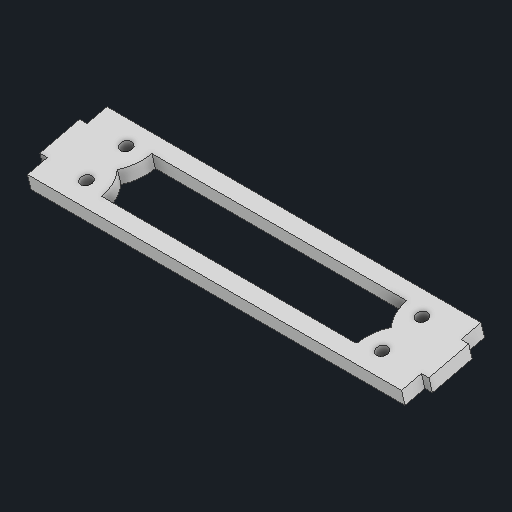
# Autodesk Inventor part: motor_mount
Saved by Autodesk Inventor 2023 (Build 270158030, 158C)
## iProperties
Created: 2022-03-25
Part Number: motor_mount
Material: Generic
Document SubType Name: Modeling
Designer: kardo
Density: 1 g/cm^3
Appearance: Default
Author: kardo
Autodesk Inventor part; units mm, degrees
ref_plane "YZ Plane" through (0, 0, 0) normal (1, 0, 0) x (0, 1, 0)
ref_plane "XZ Plane" through (0, 0, 0) normal (0, 1, 0) x (-1, 0, 0)
ref_plane "XY Plane" through (0, 0, 0) normal (0, 0, 1) x (1, 0, 0)
derived "parameters_frame.ipt"
derived "stencil_frame.ipt"
sketch "sk_cowl_joint_locations" plane through (54.6, 0, 0) normal (1, 0, 0) x (0, 1, 0)
  line L0 (-345, 16.32) -> (-262.2001, 18.586) construction
  arc A0 (-262.2001, 18.586) -> (-241.5001, 19.2432) centre (-326.8578, 2381.2399) ccw construction
  line L1 (-241.5001, 19.2432) -> (11.22, 28.376) construction
  arc A1 (36.465, 28.832) -> (11.22, 28.376) centre (36.465, -670.197) ccw construction
  line L2 (36.465, 28.832) -> (112.2, 28.832) construction
  line L3 (94.8, 30.032) -> (36.465, 30.032) construction
  arc A2 (36.465, 30.032) -> (11.1767, 29.5752) centre (36.465, -670.197) ccw construction
  line L4 (11.1767, 29.5752) -> (-241.5434, 20.4424) construction
  arc A3 (-262.2329, 19.7855) -> (-241.5434, 20.4424) centre (-326.8578, 2381.2399) ccw construction
  line L5 (-262.2329, 19.7855) -> (-345, 17.5204) construction
  line L6 (-230.0001, 3089.1136) -> (-230.0001, -1866.0023) construction
  line L7 (-114.9999, 3089.1136) -> (-114.9999, -1866.0023) construction
  line L8 (-345, 3089.1136) -> (-345, -1866.0023) construction
  line L9 (0, 3089.1136) -> (0, -1866.0023) construction
  line L10 (-230.0001, 45.0685) -> (-230.0001, 20.8596) construction
  line L11 (-114.9999, 49.9659) -> (-114.9999, 25.0155) construction
  line L12 (-345, 17.5204) -> (-345, 17.5204)
  line L13 (-345, 17.5204) -> (-345, 36.9221) construction
  line L14 (-844.2225, 3013.4797) -> (331.7536, -1884.8132) construction
  line L15 (-344.7623, 36.9221) -> (-345, 39.712) construction
  line L16 (0, 51.6) -> (0, 29.1713) construction
  line L17 (-135.791, 45.5154) -> (-130.7328, 24.4469) construction
  line L18 (-128.1079, 30.6478) -> (-131.9974, 29.714) construction
  line L19 (-130.6369, 41.1821) -> (-134.5264, 40.2483) construction
  spline S0 degree 2 poles (-345, 39.712) (-172.656, 54.3934) (0, 54.4) knots 0 0 0 1 1 1
  spline S1 degree 3 poles (0, 54.4) (37.026, 54.4) (80.784, 47.9917) (112.2, 37.536) knots 1 1 1 1 2 2 2 2
  spline S2 degree 3 poles (111.3158, 34.8793) (106.1488, 36.5989) (96.4909, 39.4217) (84.5445, 42.2265) (75.2974, 44.1359) (69.0059, 45.3094) (61.0256, 46.6466) (54.5653, 47.6105) (46.4371, 48.6777) (39.9092, 49.4192) (31.7597, 50.2005) (25.2653, 50.7072) (17.2211, 51.1873) (9.2717, 51.5118) (3.0586, 51.6) (0, 51.6) knots 1 1 1 1 1.166667 1.291667 1.333333 1.416667 1.458333 1.541667 1.583333 1.666667 1.708333 1.791667 1.833333 1.916667 2 2 2 2
  spline S3 degree 3 poles (0, 51.6) (-19.1708, 51.5993) (-52.7146, 51.3604) (-91.0402, 50.6121) (-119.7801, 49.8472) (-138.9379, 49.2354) (-162.8824, 48.3434) (-182.0358, 47.528) (-205.975, 46.3814) (-225.1241, 45.3623) (-249.0578, 43.9611) (-268.2026, 42.7383) (-292.131, 41.0825) (-316.0566, 39.2994) (-335.1942, 37.7372) (-344.7623, 36.9221) knots 0 0 0 0 0.166667 0.291667 0.333333 0.416667 0.458333 0.541666 0.583333 0.666666 0.708333 0.791666 0.833333 0.916666 1 1 1 1
  line L20 (-135.791, 45.5154) -> (-131.9015, 46.4492) construction
  line L21 (-130.7328, 24.4469) -> (-126.8434, 25.3807) construction
  line L22 (-131.9015, 46.4492) -> (-132.0904, 52.2462) construction
  point P0 (0, 0)
  point P1 (-345, 27.2213)
  point P2 (-230.0001, 32.964)
  point P3 (-114.9999, 37.4907)
  point P4 (0, 40.3857)
  point P5 (0, 40.3857)
ref_plane "plane_motor_mount" through (0, -120.75, 0) normal (0, 0.9723699, 0.2334454) x (-1, 0, 0)
ref_plane "plane_cowl_right" through (54.6, 0, 0) normal (1, 0, 0) x (0, 1, 0)
ref_plane "plane_symmetry" through (0, 0, 0) normal (1, 0, 0) x (0, 1, 0)
sketch "sk_base" plane through (0, -120.75, 0) normal (0, 0.9723699, 0.2334454) x (-1, 0, 0)
  line L0 (-54.6, -1321.492) -> (-54.6, 2983.6601) construction
  line L1 (0, -1321.492) -> (0, 2983.6601) projected
  line L2 (0, 47.7691) -> (-49.6, 47.7691)
  line L3 (-49.6, 47.7691) -> (-49.6, 42.3523)
  line L4 (-49.6, 42.3523) -> (-51.6, 42.3523)
  line L5 (-51.6, 42.3523) -> (-51.6, 31.5187)
  line L6 (-51.6, 31.5187) -> (-49.6, 31.5187)
  line L7 (-49.6, 31.5187) -> (-49.6, 26.1019)
  line L8 (-49.6, 26.1019) -> (0, 26.1019)
  point P0 (0, -28.1885)
  point P1 (-54.6, 42.3523)
  point P2 (-54.6, 31.5187)
  point P3 (-54.6, 47.7691)
  point P4 (-54.6, 26.1019)
  dimension "d2" = 5
  dimension "d3" = 2
  constraints: 14 end point, 6 point on line, 4 perpendicular, 2 parallel, 1 collinear
  measures "d2" distance between parallel lines of L0 L3
  measures "d3" distance between parallel lines of L3 L5
extrude "thicken" add sketch "sk_base" against normal blind 4
sketch "sk_cut" plane through (0, -120.75, 0) normal (0, 0.9723699, 0.2334454) x (-1, 0, 0)
  line L0 (-49.6, 26.1019) -> (0, 26.1019) construction
  line L1 (0, 26.1019) -> (0, 47.7691) projected
  line L2 (0, 47.7691) -> (-49.6, 47.7691) construction
  line L3 (-49.6, 47.7691) -> (-49.6, 42.3523) construction
  line L4 (-49.6, 42.3523) -> (-51.6, 42.3523) construction
  line L5 (-51.6, 42.3523) -> (-51.6, 31.5187) construction
  line L6 (-51.6, 31.5187) -> (-49.6, 31.5187) construction
  line L7 (-49.6, 31.5187) -> (-49.6, 26.1019) construction
  line L8 (0, 26.1019) -> (0, 47.7691) projected
  line L9 (0, 43.7691) -> (-33.8, 43.7691)
  line L10 (0, 30.1019) -> (-33.8, 30.1019)
  arc A0 (-33.8, 30.1019) -> (-36.2872, 36.9355) centre (-44.4312, 30.1019) ccw
  arc A1 (-36.2872, 36.9355) -> (-33.8, 43.7691) centre (-44.4312, 43.7691) ccw
  circle A2 centre (-39.2, 42.3691) radius 1.5
  circle A3 centre (-39.2, 31.5019) radius 1.5
  line L11 (-44.6, 47.7691) -> (-44.6, 26.1019) construction
  line L12 (-33.8, 43.7691) -> (-33.8, 30.1019) construction
  line L13 (-39.2, 31.5019) -> (-44.6, 31.5019) construction
  line L14 (-39.2, 31.5019) -> (-39.2, 26.1019) construction
  line L15 (-39.2, 42.3691) -> (-39.2, 47.7691) construction
  line L16 (-39.2, 42.3691) -> (-44.6, 42.3691) construction
  point P0 (0, -28.1885)
  point P1 (-34.4411, 33.738)
  dimension "d7" = 3
  dimension "d11" = 4
  dimension "d12" = 4
  dimension "d13" = 140
  dimension "d22" = 5
  dimension "d23" = 5.4
  dimension "d24" = 5.4
  constraints: 16 end point, 9 point on line, 5 point on circle, 4 centre point, 4 perpendicular, 3 equal length, 3 parallel, 2 equal radius, 2 line through centre
  measures "d7" diameter of A2
  measures "d11" distance between parallel lines of L2 L9
  measures "d12" distance between parallel lines of L0 L10
  measures "d22" distance between parallel lines of L11 L3
  measures "d23" distance between parallel lines of L11 L14
  measures "d24" distance between parallel lines of L14 L12
extrude "cut" cut sketch "sk_cut" along normal through all both and the other way through all
mirror "mirror" about plane through (0, 0, 0) normal (1, 0, 0)
equation "\"d2\" = cowl_liner_width"
equation "\"d3\" = bulkhead_thickness"
equation "\"d4\" = 2 * bulkhead_thickness"
equation "\"d7\" = drill_motor_mount_diam"
equation "\"d11\" = bulkhead_inset"
equation "\"d12\" = bulkhead_inset"
equation "\"d22\" = cowl_sealing_width"
equation "\"d23\" = 1.8 * drill_motor_mount_diam"
equation "\"d24\" = 1.8 * drill_motor_mount_diam"
equation "\"cowl_liner_width\" = 5"
equation "\"bulkhead_thickness\" = 2"
equation "\"drill_motor_mount_diam\" = 3"
equation "\"bulkhead_inset\" = 4"
equation "\"cowl_sealing_width\" = 5"
body "Solid1"
